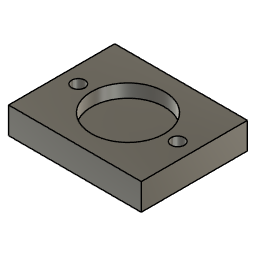
Beginning V1 (Autodesk Fusion 360 design; units mm, degrees)
Autodesk Fusion 360 part; units mm, degrees
sketch "Sketch1" plane through (0, 0, 0) normal (0, 0, 1) x (1, 0, 0)
  line L0 (50, 40) -> (-50, 40)
  line L1 (-50, 40) -> (-50, -40)
  line L2 (-50, -40) -> (50, -40)
  line L3 (50, -40) -> (50, 40)
  line L4 (50, 40) -> (-50, -40) construction
  line L5 (-50, 40) -> (50, -40) construction
  line L6 (-50, 0) -> (50, 0) construction
  line L7 (0, 46.7573) -> (0, -57.5987) construction
  circle A0 centre (-37.5, 0) radius 5
  circle A1 centre (37.5, 0) radius 5
  dimension "d1" = 100
  dimension "d2" = 80
  dimension "d3" = 10
  dimension "d4" = 75
  constraint horizontal L0
  constraint perpendicular L0 L1
  constraint parallel L0 L2
  constraint parallel L1 L3
  constraint coincident L4 origin
  constraint coincident L5 origin
  constraint midpoint L1 L6.start
  constraint midpoint L3 L6.end
  constraint symmetric L1 L3 L7
  constraint coincident L6 A0.centre
  constraint symmetric L7 A0 A1
  measures "d1" distance of L1.end L2.end
  measures "d2" distance of L0.end L1.end
  measures "d3" diameter of A0
  measures "d4" distance of A0.centre A1.centre
extrude "Extrude1" add sketch "Sketch1" along normal blind 25
extrude "Extrude2" cut 1 faces at (11.2782, -27.8003, 25) along direction (0, 0, -1) blind 5
sketch "Sketch2" plane through (0, 0, 20) normal (0, 0, 1) x (-1, 0, 0)
  circle A0 centre (37.5, 0) radius 5
  circle A1 centre (-37.5, 0) radius 5
  line L0 (-50, 40) -> (-50, -40)
  line L1 (-50, -40) -> (50, -40)
  line L2 (50, -40) -> (50, 40)
  line L3 (50, 40) -> (-50, 40)
  circle A2 centre (0, 0) radius 27.5
  dimension "d9" = 55
  constraint coincident A2.centre origin
  measures "d9" diameter of A2
extrude "Extrude3" cut sketch "Sketch2" against normal blind 10 contours A2
